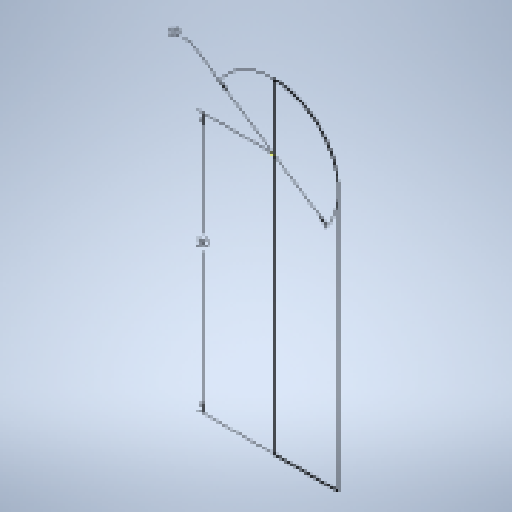
# Autodesk Inventor part: BeltClamp
Saved by Autodesk Inventor 2023 (Build 270158000, 158)
## iProperties
Created: 2023-08-18
Part Number: BeltClamp
Material: Generic
Document SubType Name: Modeling
Designer: Felix
Density: 1 g/cm^3
Appearance: Default
Author: Felix
Autodesk Inventor part; units mm, degrees
ref_plane "YZ Plane" through (0, 0, 0) normal (1, 0, 0) x (0, 1, 0)
ref_plane "XZ Plane" through (0, 0, 0) normal (0, 1, 0) x (-1, 0, 0)
ref_plane "XY Plane" through (0, 0, 0) normal (0, 0, 1) x (1, 0, 0)
sketch "Sketch1" plane through (0, 0, 0) normal (0, 0, 1) x (1, 0, 0)
  arc A0 (5, 0) -> (0, 5) centre (0, 0) ccw
  line L0 (0, 0) -> (0, -20)
  line L1 (0, -20) -> (5, -20)
  line L2 (5, -20) -> (5, 0)
  line L3 (0, 0) -> (0, 5)
  arc A1 (6.3, -0.5) -> (6.3, -1.5) centre (6.3, -1) ccw
  line L4 (6.3, -0.5) -> (6.5, -0.5)
  line L5 (6.3, -1.5) -> (6.5, -1.5)
  line L6 (6.5, 0) -> (6.5, -0.5)
  line L7 (6.5, -1.5) -> (6.5, -2)
  arc A2 (6.3, -2.5) -> (6.3, -3.5) centre (6.3, -3) ccw
  line L8 (6.3, -2.5) -> (6.5, -2.5)
  line L9 (6.3, -3.5) -> (6.5, -3.5)
  line L10 (6.5, -2) -> (6.5, -2.5)
  line L11 (6.5, -3.5) -> (6.5, -4)
  arc A3 (6.3, -4.5) -> (6.3, -5.5) centre (6.3, -5) ccw
  line L12 (6.3, -4.5) -> (6.5, -4.5)
  line L13 (6.3, -5.5) -> (6.5, -5.5)
  line L14 (6.5, -4) -> (6.5, -4.5)
  line L15 (6.5, -5.5) -> (6.5, -6)
  arc A4 (6.3, -6.5) -> (6.3, -7.5) centre (6.3, -7) ccw
  line L16 (6.3, -6.5) -> (6.5, -6.5)
  line L17 (6.3, -7.5) -> (6.5, -7.5)
  line L18 (6.5, -6) -> (6.5, -6.5)
  line L19 (6.5, -7.5) -> (6.5, -8)
  arc A5 (6.3, -8.5) -> (6.3, -9.5) centre (6.3, -9) ccw
  line L20 (6.3, -8.5) -> (6.5, -8.5)
  line L21 (6.3, -9.5) -> (6.5, -9.5)
  line L22 (6.5, -8) -> (6.5, -8.5)
  line L23 (6.5, -9.5) -> (6.5, -10)
  arc A6 (6.3, -10.5) -> (6.3, -11.5) centre (6.3, -11) ccw
  line L24 (6.3, -10.5) -> (6.5, -10.5)
  line L25 (6.3, -11.5) -> (6.5, -11.5)
  line L26 (6.5, -10) -> (6.5, -10.5)
  line L27 (6.5, -11.5) -> (6.5, -12)
  arc A7 (6.3, -12.5) -> (6.3, -13.5) centre (6.3, -13) ccw
  line L28 (6.3, -12.5) -> (6.5, -12.5)
  line L29 (6.3, -13.5) -> (6.5, -13.5)
  line L30 (6.5, -12) -> (6.5, -12.5)
  line L31 (6.5, -13.5) -> (6.5, -14)
  arc A8 (6.3, -14.5) -> (6.3, -15.5) centre (6.3, -15) ccw
  line L32 (6.3, -14.5) -> (6.5, -14.5)
  line L33 (6.3, -15.5) -> (6.5, -15.5)
  line L34 (6.5, -14) -> (6.5, -14.5)
  line L35 (6.5, -15.5) -> (6.5, -16)
  arc A9 (6.3, -16.5) -> (6.3, -17.5) centre (6.3, -17) ccw
  line L36 (6.3, -16.5) -> (6.5, -16.5)
  line L37 (6.3, -17.5) -> (6.5, -17.5)
  line L38 (6.5, -16) -> (6.5, -16.5)
  line L39 (6.5, -17.5) -> (6.5, -18)
  arc A10 (6.3, -18.5) -> (6.3, -19.5) centre (6.3, -19) ccw
  line L40 (6.3, -18.5) -> (6.5, -18.5)
  line L41 (6.3, -19.5) -> (6.5, -19.5)
  line L42 (6.5, -18) -> (6.5, -18.5)
  line L43 (6.5, -19.5) -> (6.5, -20)
  arc A11 (6.3, -20.5) -> (6.3, -21.5) centre (6.3, -21) ccw
  line L44 (6.3, -20.5) -> (6.5, -20.5)
  line L45 (6.3, -21.5) -> (6.5, -21.5)
  line L46 (6.5, -20) -> (6.5, -20.5)
  line L47 (6.5, -21.5) -> (6.5, -22)
  arc A12 (6.3, -22.5) -> (6.3, -23.5) centre (6.3, -23) ccw
  line L48 (6.3, -22.5) -> (6.5, -22.5)
  line L49 (6.3, -23.5) -> (6.5, -23.5)
  line L50 (6.5, -22) -> (6.5, -22.5)
  line L51 (6.5, -23.5) -> (6.5, -24)
  arc A13 (6.3, -24.5) -> (6.3, -25.5) centre (6.3, -25) ccw
  line L52 (6.3, -24.5) -> (6.5, -24.5)
  line L53 (6.3, -25.5) -> (6.5, -25.5)
  line L54 (6.5, -24) -> (6.5, -24.5)
  line L55 (6.5, -25.5) -> (6.5, -26)
  arc A14 (6.3, -26.5) -> (6.3, -27.5) centre (6.3, -27) ccw
  line L56 (6.3, -26.5) -> (6.5, -26.5)
  line L57 (6.3, -27.5) -> (6.5, -27.5)
  line L58 (6.5, -26) -> (6.5, -26.5)
  line L59 (6.5, -27.5) -> (6.5, -28)
  arc A15 (6.3, -28.5) -> (6.3, -29.5) centre (6.3, -29) ccw
  line L60 (6.3, -28.5) -> (6.5, -28.5)
  line L61 (6.3, -29.5) -> (6.5, -29.5)
  line L62 (6.5, -28) -> (6.5, -28.5)
  line L63 (6.5, -29.5) -> (6.5, -30)
  line L64 (6.5, 0) -> (11.5, 0)
  line L65 (11.5, 0) -> (11.5, -30)
  line L66 (11.5, -30) -> (6.5, -30)
  dimension "d0" = 10
  dimension "d15" = 20
  dimension "d22" = 1
  dimension "d23" = 2
  dimension "d25" = 0.2
  dimension "d26" = 0.5
  dimension "d27" = 0.5
  dimension "d28" = 1.5
  dimension "d31" = 2
  dimension "d36" = 5
  constraints: 134 end point, 32 point on circle, 16 centre point, 15 point on line, 8 perpendicular, 5 vertical, 3 tangent, 1 coincident, 1 collinear, 1 horizontal, 1 horizontal alignment, 167 other
  measures "d0" diameter of A0
  measures "d15" distance from line of point (0, 0) L1
  measures "d22" diameter of A1
  measures "d23" distance of L6.start L7.end
  measures "d25" distance from line of L7 A1.centre
  measures "d26" distance from line of L6.start L4
  measures "d27" distance of L5.end L7.end
  measures "d28" distance between parallel lines of L2 L7
  measures "d31" distance of A1.centre A2.centre
  measures "d36" distance of L6.start L64.end
extrude "Extrusion1" add sketch "Sketch1" along normal blind 12
equation "\"d26\" = d27"
body "Solid1"
